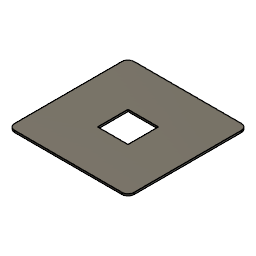
core-p1_stencil_jig (Autodesk Fusion 360 design; units mm, degrees)
part number: 2025-12-29-13-24-03-887
Autodesk Fusion 360 part; units mm, degrees
sketch "Sketch1" plane through (0, 0, 0) normal (0, 1, 0) x (1, 0, 0)
  line L0 (0, 0) -> (25.3, 0)
  line L1 (25.3, 0) -> (25.3, 25.3)
  line L2 (25.3, 25.3) -> (0, 25.3)
  line L3 (0, 25.3) -> (0, 0)
  line L4 (-32.35, 62.65) -> (57.65, 62.65)
  line L5 (62.65, 57.65) -> (62.65, -32.35)
  line L6 (57.65, -37.35) -> (-32.35, -37.35)
  line L7 (-37.35, -32.35) -> (-37.35, 57.65)
  arc A0 (-32.35, 62.65) -> (-37.35, 57.65) centre (-32.35, 57.65) ccw
  arc A1 (62.65, 57.65) -> (57.65, 62.65) centre (57.65, 57.65) ccw
  arc A2 (57.65, -37.35) -> (62.65, -32.35) centre (57.65, -32.35) ccw
  arc A3 (-37.35, -32.35) -> (-32.35, -37.35) centre (-32.35, -32.35) ccw
  point P0 (-37.35, 62.65)
  point P1 (62.65, 62.65)
  point P2 (62.65, -37.35)
  dimension "d1" = 25.3
  dimension "d2" = 25.3
  dimension "d3" = 100
  dimension "d4" = 100
  dimension "d5" = 37.35
  dimension "d6" = 37.35
  dimension "d7" = 5
  dimension "d8" = 5
  constraint horizontal L0
  constraint vertical L1
  constraint horizontal L2
  constraint vertical L3
  constraint coincident L0.start L3.end
  constraint horizontal L4
  constraint vertical L5
  constraint horizontal L6
  constraint vertical L7
  constraint coincident P0 L4
  constraint coincident P0 L7
  constraint tangent L4 A0
  constraint tangent L7 A0
  constraint coincident P1 L4
  constraint coincident P1 L5
  constraint tangent L4 A1
  constraint tangent L5 A1
  constraint coincident P2 L5
  constraint coincident P2 L6
  constraint tangent L5 A2
  constraint tangent L6 A2
  constraint equal A1 A2
  constraint tangent L6 A3
  constraint tangent L7 A3
  constraint equal A1 A3
  measures "d1" distance of L0.start L0.end
  measures "d2" distance of L0.start L2.end
  measures "d3" distance of P0 P1
  measures "d4" distance of P1 P2
  measures "d5" distance of L2 L4
  measures "d6" distance of L3 L7
  measures "d7" radius of A0
  measures "d8" radius of A1
extrude "Extrude1" add sketch "Sketch1" along normal blind 1.54
equation "d5 = ( ( 100 - 25.3 ) / 2 ) * 1 mm"
equation "d6 = ( ( 100 - 25.3 ) / 2 ) * 1 mm"
